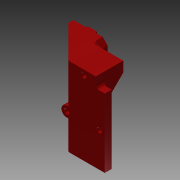
# Autodesk Inventor part: stopclamp
Saved by Autodesk Inventor 2015 SP1 (Build 190203100, 203)
## iProperties
Created: 2015-02-07
Part Number: stopclamp
Material: Generic
Document SubType Name: Modeling
Designer: Joseph
Density: 1 g/cm^3
Appearance: Red
Author: Joseph
Autodesk Inventor part; units mm, degrees
note: some values were not read from the file. Chosen so that the rebuilt part matches the saved one: edges of "Fillet4".
ref_plane "YZ Plane" through (0, 0, 0) normal (1, 0, 0) x (0, 1, 0)
ref_plane "XZ Plane" through (0, 0, 0) normal (0, 1, 0) x (-1, 0, 0)
ref_plane "XY Plane" through (0, 0, 0) normal (0, 0, 1) x (1, 0, 0)
sketch "Sketch1" plane through (0, 0, 0) normal (0, 0, 1) x (1, 0, 0)
  point P0 (0, 0)
sketch "Sketch2" plane through (0, 0, 0) normal (0, 0, 1) x (1, 0, 0)
  line L0 (10, 20) -> (-10, 20)
  line L1 (-10, 20) -> (-10, -20)
  line L2 (-10, -20) -> (10, -20)
  line L3 (10, -20) -> (10, 20)
  line L4 (10, 20) -> (-10, -20) construction
  line L5 (-10, 20) -> (10, -20) construction
  point P0 (0, 0)
  dimension "d0" = 20
  dimension "d1" = 40
  constraints: 12 end point, 2 midpoint, 2 parallel, 1 horizontal, 1 perpendicular
  measures "d0" distance of L2.end L1.end
  measures "d1" distance of L1.end L0.end
extrude "Extrusion1" add sketch "Sketch2" along normal blind 3
sketch "Sketch9" plane through (-10, 20, 0) normal (0, 1, 0) x (1, 0, 0)
  line L0 (-9.5711, -3) -> (42.6862, -3) construction
  line L1 (0, -3) -> (24.4142, -27.4142)
  line L2 (0, -3) -> (34.5269, -3) construction
  line L3 (25.8284, -28) -> (46.2473, -28)
  line L4 (46.2473, -24) -> (46.2473, -28)
  line L5 (46.2473, -24) -> (31.8654, -24)
  line L6 (31.8654, -24) -> (20, -3)
  line L7 (0, -3) -> (20, -3)
  arc A0 (24.4142, -27.4142) -> (25.8284, -28) centre (25.8284, -26) ccw
  point P0 (10, 0)
  point P1 (25, -28)
  dimension "d35" = 45
  dimension "d40" = 4
  dimension "d41" = 25
  constraints: 16 end point, 3 horizontal, 3 point on line, 2 point on circle, 2 tangent, 1 centre point, 1 collinear, 1 equal length
  measures "d35" angle of L1 L2
  measures "d40" distance of L4.start L3.end
  measures "d41" distance between parallel lines of L3 L2
extrude "Extrusion6" add sketch "Sketch9" against normal up to surface (40 mm away)
sketch "Sketch3" plane through (15.8284, 20, 28) normal (0, 0, 1) x (1, 0, 0)
  circle A0 centre (-15.8284, -20) radius 10 construction
  line L0 (20.4188, 0) -> (20.4188, -40) projected
  line L1 (20.4188, -20) -> (-22.019, -20) construction
  line L2 (-5.8284, 0) -> (-25.8284, 0) construction
  line L3 (-25.8284, -40) -> (-5.8284, -40) construction
  line L4 (-15.8284, 0) -> (-15.8284, -40) construction
  point P0 (-15.8284, -10)
  point P1 (-15.8383, -30)
  dimension "d4" = 20
  constraints: 4 end point, 4 midpoint, 2 point on circle, 1 centre point, 1 horizontal, 1 point on line
  measures "d4" diameter of A0
hole "Hole1" at (0, 10, 28) at (-0.0098, -10, 28) direction (0, 0, -1) diameter 4.5 end through all counterbore diameter 8 counterbore depth 25 clearance for "Socket Head Cap Screw" size "M4" standard "Ansi Metric M Profile"
sketch "Sketch4" plane through (15.8284, 20, 28) normal (0, 0, 1) x (1, 0, 0)
  circle A0 centre (-15.8284, -10) radius 2.25
  circle A1 centre (-15.8284, -30) radius 2.25
  circle A2 centre (-15.8284, -10) radius 4.5 construction
  circle A3 centre (-15.8284, -30) radius 4.5 construction
  line L0 (0, -40) -> (20.4188, -40) projected
  line L1 (20.4188, 0) -> (20.4188, -40) projected
  line L2 (0, 0) -> (20.4188, 0) projected
  line L3 (0, 0) -> (0, -40) projected
  line L4 (20.4188, -20) -> (-21.8157, -20) construction
  line L5 (-5.8284, 0) -> (-25.8284, 0) construction
  line L6 (-25.8284, -40) -> (-5.8284, -40) construction
  line L7 (-15.8284, 0) -> (-15.8284, -40) construction
  circle A4 centre (-15.8284, -20) radius 10 construction
  dimension "d12" = 9
  dimension "d13" = 9
  dimension "d39" = 20
  constraints: 5 centre point, 4 end point, 4 midpoint, 2 coincident, 2 point on circle, 2 point on line, 1 horizontal
  measures "d12" diameter of A2
  measures "d13" diameter of A3
  measures "d39" diameter of A4
sketch "Sketch5" plane through (0, 0, 0) normal (0, 0, -1) x (-1, 0, 0)
  circle A0 centre (0, 10) radius 2.25 projected
  circle A1 centre (0.0098, -10) radius 2.25 projected
  line L0 (-2.7671, 20.001) -> (2.7334, 20.001)
  line L1 (2.7668, -19.999) -> (-2.7332, -19.999)
  line L2 (-2.7671, 20.001) -> (2.7668, -19.999) construction
  line L3 (2.7334, 20.001) -> (-2.7332, -19.999) construction
  line L4 (2.75, 6.875) -> (-2.75, 6.875)
  line L5 (-2.7671, 13.126) -> (2.7334, 13.126)
  line L6 (2.75, 7.25) -> (-3.125, 13.125) construction
  line L7 (-3.125, 6.875) -> (3.125, 13.125) construction
  line L8 (2.7668, -13.124) -> (-2.7332, -13.124)
  line L9 (-2.75, -6.875) -> (2.75, -6.875)
  line L10 (1.604, -11.5942) -> (-3.1152, -6.875) construction
  line L11 (-3.1152, -13.125) -> (3.1348, -6.875) construction
  line L12 (2.7334, 20.001) -> (2.7334, 13.126)
  line L13 (-2.7671, 13.126) -> (-2.7671, 20.001)
  line L14 (-2.7332, -19.999) -> (-2.7332, -13.124)
  line L15 (-2.75, -6.875) -> (-2.75, 6.875)
  line L16 (2.75, 6.875) -> (2.75, -6.875)
  line L17 (2.7668, -13.124) -> (2.7668, -19.999)
  point P0 (0, 0)
  dimension "d14" = 5.5
  dimension "d15" = 40
  dimension "d16" = 6.25
  dimension "d17" = 6.25
  dimension "d18" = 6.25
  dimension "d19" = 6.25
  constraints: 36 end point, 12 parallel, 5 point on line, 3 horizontal, 3 perpendicular, 2 midpoint
  measures "d14" distance of L1.start L1.end
  measures "d15" distance of L0.end L1.start
  measures "d16" distance of L6.end L7.end
  measures "d17" distance of L7.start L6.end
  measures "d18" distance of L10.end L11.end
  measures "d19" distance of L11.start L10.end
extrude "Extrusion2" add sketch "Sketch5" along normal blind 1 contours L0 L12 L5 L13 | L1 L14 L8 L17 | L16 L9 L15 L4
sketch "Sketch10" plane through (36.2473, 20, 24) normal (0, 0, -1) x (-1, 0, 0)
  line L0 (14.3819, 0) -> (14.3819, -40) projected
  line L1 (49.8819, -14) -> (-21.1181, -14)
  line L2 (-21.1181, -14) -> (-21.1181, -26)
  line L3 (-21.1181, -26) -> (49.8819, -26)
  line L4 (49.8819, -26) -> (49.8819, -14)
  line L5 (49.8819, -14) -> (-21.1181, -26) construction
  line L6 (-21.1181, -14) -> (49.8819, -26) construction
  point P0 (36.2473, -20)
  point P1 (14.3819, -20)
  dimension "d42" = 71
  dimension "d43" = 12
  constraints: 12 end point, 3 midpoint, 2 parallel, 1 horizontal, 1 perpendicular
  measures "d42" distance of L3.end L2.end
  measures "d43" distance of L2.end L1.end
extrude "Extrusion7" cut sketch "Sketch10" along normal blind 8
sketch "Sketch11" plane through (11, 6, 24) normal (0, -1, 0) x (1, 0, 0)
  line L0 (-8, -8) -> (6.3452, -8) projected
  line L1 (6.3452, -8) -> (-1, -21)
  line L2 (-1, -21) -> (-8, -8)
  line L3 (6.3452, -8) -> (-8, -8)
  point P0 (-11, -24)
  constraints: 6 end point
extrude "Extrusion8" cut sketch "Sketch11" along normal up to surface (12 mm away) from surface at 0
fillet "Fillet1" radius 2 1 edges at (3, 0, 16)
sketch "Sketch12" plane through (15.8284, 20, 28) normal (0, 0, 1) x (1, 0, 0)
  circle A0 centre (17.1141, -20.1309) radius 1.535 projected
  circle A1 centre (-1.8159, -20.1309) radius 1.535 projected
  point P0 (-15.8284, -20)
  constraints: 2 coincident
hole "Hole2" at (14.0125, -0.1309, 28) at (32.9425, -0.1309, 28) direction (0, 0, -1) diameter 3 end through all clearance for "Socket Head Cap Screw" size "M3" standard "Ansi Metric M Profile"
sketch "Sketch13" plane through (15.8284, 20, 28) normal (0, 0, 1) x (1, 0, 0)
  circle A0 centre (17.1141, -20.1309) radius 1.5 projected
  circle A1 centre (-1.8159, -20.1309) radius 1.535 projected
  line L0 (17.1141, -20.1309) -> (-1.8159, -20.1309) construction
  line L1 (17.1141, -17.1155) -> (-1.8159, -17.1155)
  line L2 (-1.8159, -23.1463) -> (17.1141, -23.1463)
  arc A2 (17.1141, -23.1463) -> (17.1141, -17.1155) centre (17.1141, -20.1309) ccw
  arc A3 (-1.8159, -17.1155) -> (-1.8159, -23.1463) centre (-1.8159, -20.1309) ccw
  line L3 (-4.8284, -14) -> (-4.8284, -26) projected
  point P0 (-15.8284, -20)
  point P1 (7.6491, -20.1309)
  point P2 (-4.8284, -20)
  constraints: 8 end point, 5 point on circle, 4 tangent, 2 centre point, 2 midpoint, 1 horizontal, 1 parallel
extrude "Extrusion9" add sketch "Sketch13" against normal up to surface (4 mm away) from surface at 0
sketch "Sketch15" plane through (11, 20, 24) normal (0, 1, 0) x (-1, 0, 0)
  line L0 (-20, 4) -> (-4.8284, 4)
  line L1 (12, -12) -> (-20, -12)
  line L2 (-20, -12) -> (-20, 4)
  line L3 (1, -24) -> (8.2329, -24) projected
  line L4 (21, -21) -> (-3.4142, 3.4142) projected
  arc A0 (-3.4142, 3.4142) -> (-4.8284, 4) centre (-4.8284, 2) ccw projected
  line L5 (-4.8284, 4) -> (-25.2473, 4) projected
  point P0 (0, 0)
  point P1 (12.75, 4)
  point P2 (7, -12)
  point P3 (7, -7)
  dimension "d60" = 32
  dimension "d82" = 12
  constraints: 6 end point, 5 point on line, 1 horizontal, 1 parallel, 1 perpendicular, 1 point on circle
  measures "d60" distance of L1.start L1.end
  measures "d82" distance between parallel lines of L1 L3
extrude "Extrusion11" add sketch "Sketch15" along normal blind 6
sketch "Sketch16" plane through (15, 20, 28) normal (0, 0, 1) x (-1, 0, 0)
  line L0 (-0.8284, -6) -> (-16, -6) projected
  line L1 (-16, 0) -> (-21.2473, 0) projected
  line L2 (10, -6) -> (10, 0) construction
  line L3 (27.2526, -3) -> (5.5607, -3) construction
  line L4 (-9, 0) -> (-9, -6) construction
  line L5 (-16, 0) -> (-16, -6) projected
  point P0 (23.5391, 0)
  point P1 (28, 0)
  point P2 (0, 6)
  point P3 (0, 0)
  point P4 (14.5715, 0)
  point P5 (15, 20)
  point P6 (10, -3)
  point P7 (-9, -3)
  point P8 (12, -6)
  point P9 (2, 0)
  point P10 (1, 0)
  point P11 (14, -3)
  dimension "d69" = 19
  dimension "d95" = 7
  constraints: 6 end point, 4 point on line, 2 midpoint, 2 vertical, 1 horizontal, 3 other
  measures "d69" distance between parallel lines of L4 L2
  measures "d95" distance between parallel lines of L5 L4
hole "Hole3" at (5, 23, 28) at (24, 23, 28) direction (0, 0, -1) diameter 3 end through all clearance for "Socket Head Cap Screw" size "M3" standard "Ansi Metric M Profile"
sketch "Sketch18" plane through (36.2473, 20, 24) normal (0, 0, -1) x (-1, 0, 0)
  arc A0 (25.2473, -20.2618) -> (25.2473, -20) centre (22.2347, -20.1309) ccw projected
  circle A1 centre (3.3047, -20.1309) radius 1.5 projected
  line L0 (17.7697, -25.1309) -> (7.7697, -25.1309)
  line L1 (7.7697, -25.1309) -> (7.7697, -15.1309)
  line L2 (7.7697, -15.1309) -> (17.7697, -15.1309)
  line L3 (17.7697, -15.1309) -> (17.7697, -25.1309)
  line L4 (17.7697, -25.1309) -> (7.7697, -15.1309) construction
  line L5 (7.7697, -25.1309) -> (17.7697, -15.1309) construction
  line L6 (22.2347, -20.1309) -> (3.3047, -20.1309) construction
  point P0 (36.2473, -20)
  point P1 (12.7697, -20.1309)
  dimension "d83" = 10
  dimension "d84" = 10
  constraints: 14 end point, 3 midpoint, 2 horizontal, 2 parallel, 1 perpendicular
  measures "d83" distance of L1.end L2.end
  measures "d84" distance of L0.end L1.end
extrude "Extrusion12" cut sketch "Sketch18" against normal blind 1.5 contours L0 L1 L2 L3
chamfer "Chamfer1" distance 1.5 angle 45 4 edges at (23.4775, -5.1309, 25.5) (18.4775, -0.1309, 25.5) (23.4775, 4.8691, 25.5) (28.4775, -0.1309, 25.5)
chamfer "Chamfer2" distance 3 angle 45 2 edges at (12.5426, 20, 7.5) (10, 20, 1.5)
chamfer "Chamfer3" distance 12 angle 45 1 edges at (26.4327, 20, 24)
sketch "Sketch19" plane through (36.2473, -20, 24) normal (0, 0, -1) x (-1, 0, 0)
  line L0 (7.7697, 24.8691) -> (17.7697, 24.8691) projected
  line L1 (11.0197, 9.7382) -> (14.5197, 9.7382)
  line L2 (14.5197, 9.7382) -> (14.5197, 40)
  line L3 (14.5197, 40) -> (11.0197, 40)
  line L4 (11.0197, 40) -> (11.0197, 9.7382)
  line L5 (11.0197, 9.7382) -> (14.5197, 40) construction
  line L6 (14.5197, 9.7382) -> (11.0197, 40) construction
  point P0 (36.2473, 20)
  point P1 (12.7697, 24.8691)
  dimension "d102" = 3.5
  constraints: 12 end point, 3 midpoint, 2 parallel, 1 horizontal, 1 perpendicular
  measures "d102" distance of L1.start L1.end
extrude "Extrusion13" cut sketch "Sketch19" along normal up to surface (12 mm away)
fillet "Fillet4" radius 2 5 edges at (18.4064, 14.122, 17.8781) (31, 14, 24) (2.8039, 6, 14.6638) (7.1372, 6, 8.3166) (31, 20, 26)
body "Solid1"
